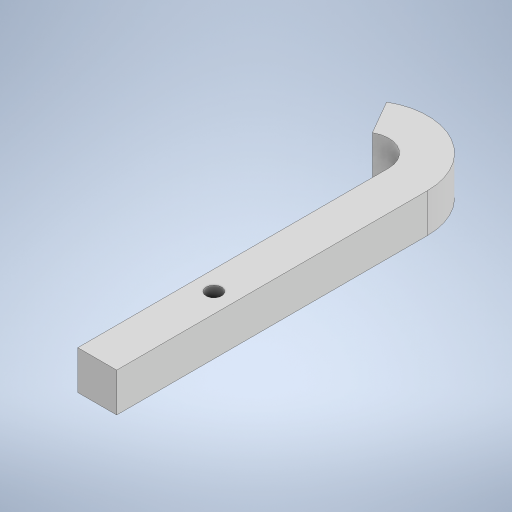
# Autodesk Inventor part: atividade_14A_garra
Saved by Autodesk Inventor 2024.2 (Build 282272000, 272)
## iProperties
Created: 2024-03-04
Part Number: atividade_14A_garra
Material: Generic
Document SubType Name: Modeling
Designer: 082220042
Density: 1 g/cm^3
Appearance: Default
Author: 082220042
Autodesk Inventor part; units mm, degrees
ref_plane "YZ Plane" through (0, 0, 0) normal (1, 0, 0) x (0, 1, 0)
ref_plane "XZ Plane" through (0, 0, 0) normal (0, 1, 0) x (-1, 0, 0)
ref_plane "XY Plane" through (0, 0, 0) normal (0, 0, 1) x (1, 0, 0)
sketch "Sketch1" plane through (0, 0, 0) normal (0, 1, 0) x (-1, 0, 0)
  line L0 (0, 0) -> (15, 0)
  line L1 (15, 0) -> (15, -120)
  line L2 (0, -120) -> (0, 0)
  arc A0 (0, -120) -> (37.5, -141.6506) centre (25, -120) ccw
  arc A1 (15, -120) -> (30, -128.6603) centre (25, -120) ccw
  line L3 (30, -128.6603) -> (37.5, -141.6506)
  line L4 (25, -120) -> (75, -120) construction
  circle A2 centre (7.5, -45) radius 3
  dimension "d1" = 120
  dimension "d9" = 20
  dimension "d11" = 60
  dimension "d12" = 15
  dimension "d13" = 6
  dimension "d14" = 45
  dimension "d15" = 7.5
  constraints: 10 end point, 4 point on circle, 3 centre point, 2 horizontal, 1 coincident, 1 parallel, 1 perpendicular, 1 point on line
  measures "d1" distance of L0.end L1.end
  measures "d9" diameter of A1
  measures "d11" angle of L3 L4
  measures "d12" distance of L3.start L3.end
  measures "d13" diameter of A2
  measures "d14" distance from line of L0 A2.centre
  measures "d15" distance from line of L2 A2.centre
extrude "Extrusion1" add sketch "Sketch1" along normal blind 15
body "Solid1"
